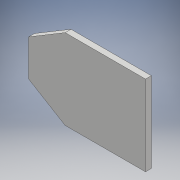
# Autodesk Inventor part: Foot
Saved by Autodesk Inventor 2018 (Build 220112000, 112)
## iProperties
Created: 2018-04-22
Part Number: Foot
Material: Generic
Document SubType Name: Modeling
Designer: HP
Density: 1 g/cm^3
Appearance: Default
Mass: 7.83375 g
Surface Area: 82.9037 cm^2
Volume: 7.83375 cm^3
Author: HP
Autodesk Inventor part; units mm, degrees
ref_plane "YZ Plane" through (0, 0, 0) normal (1, 0, 0) x (0, 1, 0)
ref_plane "XZ Plane" through (0, 0, 0) normal (0, 1, 0) x (-1, 0, 0)
ref_plane "XY Plane" through (0, 0, 0) normal (0, 0, 1) x (1, 0, 0)
sketch "Sketch1" plane through (0, 0, 0) normal (0, 1, 0) x (-1, 0, 0)
  line L0 (0, 0) -> (80, 0)
  line L1 (80, 0) -> (80, -55)
  line L2 (80, -55) -> (0, -55)
  line L3 (0, -55) -> (0, 0)
  dimension "d0" = 80
  dimension "d1" = 55
  constraints: 8 end point, 2 parallel, 1 horizontal, 1 perpendicular
  measures "d0" distance of L1.end L2.end
  measures "d1" distance of L0.end L1.end
extrude "Extrusion1" add sketch "Sketch1" along normal blind 4
sketch "Sketch9" plane through (0, 4, 0) normal (0, 1, 0) x (1, 0, 0)
  line L0 (-80, 0) -> (0, 0) projected
  line L1 (-80, 55) -> (-80, 0) projected
  line L2 (-55, 0) -> (-80, 0)
  line L3 (-80, 0) -> (-80, 15)
  line L4 (-80, 15) -> (-55, 0)
  line L5 (0, 55) -> (-80, 55) projected
  line L6 (-55, 55) -> (-80, 55)
  line L7 (-80, 55) -> (-80, 40)
  line L8 (-80, 40) -> (-55, 55)
  dimension "d11" = 15
  dimension "d12" = 15
  dimension "d37" = 25
  dimension "d38" = 25
  constraints: 12 end point, 4 point on line, 1 collinear, 1 perpendicular
  measures "d11" distance of L0.start L3.end
  measures "d12" distance of L1.start L7.end
  measures "d37" distance of L1.start L6.start
  measures "d38" distance of L0.start L2.start
extrude "Extrusion4" cut sketch "Sketch9" against normal blind 4
shell "Shell1" thickness 2 removed faces 1 at (-18.3333, 4, -18.3333)
body "Solid1"
